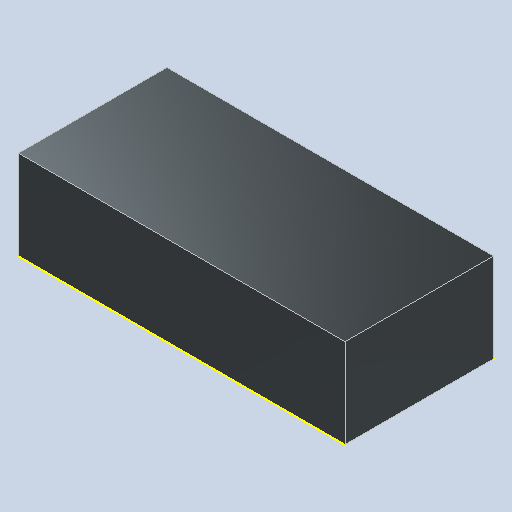
# Autodesk Inventor part: brick
Saved by Autodesk Inventor 2023 (Build 270158000, 158)
## iProperties
Created: 2022-10-04
Part Number: brick
Material: Iron, Gray
Document SubType Name: Modeling
Designer: carso
Density: 7.15 g/cm^3
Appearance: Iron Gray
Author: carso
Autodesk Inventor part; units mm, degrees
ref_plane "YZ Plane" through (0, 0, 0) normal (1, 0, 0) x (0, 1, 0)
ref_plane "XZ Plane" through (0, 0, 0) normal (0, 1, 0) x (-1, 0, 0)
ref_plane "XY Plane" through (0, 0, 0) normal (0, 0, 1) x (1, 0, 0)
sketch "Sketch1" plane through (0, 0, 0) normal (0, 1, 0) x (-1, 0, 0)
  line L0 (0, 0) -> (110, 0)
  line L1 (110, 0) -> (110, 50)
  line L2 (110, 50) -> (0, 50)
  line L3 (0, 50) -> (0, 0)
  dimension "d0" = 110
  dimension "d1" = 50
  constraints: 8 end point, 2 parallel, 1 horizontal, 1 perpendicular
  measures "d0" distance of L2.end L1.end
  measures "d1" distance of L0.end L1.end
extrude "Extrusion1" add sketch "Sketch1" along normal blind 30
sketch "Sketch2" plane through (0, 0, 0) normal (0, -1, 0) x (1, 0, 0)
  line L0 (-110, 50) -> (0, 50) projected
  line L1 (-55, 50) -> (-55, 0)
  line L2 (0, 0) -> (-110, 0) projected
  constraints: 2 end point, 2 midpoint
body "Solid1"
